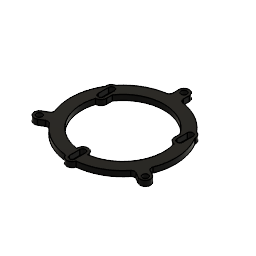
Mirror Mount Part 1 v1 (Autodesk Fusion 360 design; units mm, degrees)
Autodesk Fusion 360 part; units mm, degrees
note: some values were not read from the file. Set by a fixed rule: which sketch regions a step uses.
sketch "Sketch1" plane through (0, 0, 0) normal (0, 1, 0) x (1, 0, 0)
  circle A0 centre (0, 0) radius 26
  line L0 (0, 0) -> (22.5167, 13)
  line L1 (0, 0) -> (26, 0) construction
  line L2 (0, 0) -> (-22.5167, 13)
  line L3 (0, 0) -> (26, 0) construction
  line L4 (0, 0) -> (0, -26)
  circle A1 centre (0, 0) radius 23.5
  circle A2 centre (0, 0) radius 28.5
  line L5 (-22.5167, 13) -> (-22.5167, 16)
  line L6 (-22.5167, 13) -> (-22.5167, 10)
  line L7 (-24.1667, 10) -> (-24.1667, 16)
  line L8 (-20.8667, 10) -> (-20.8667, 16)
  line L9 (0, -26) -> (0, -23)
  line L10 (0, -26) -> (0, -29)
  line L11 (0, -26) -> (0, -23)
  line L12 (0, -29) -> (-1.65, -29)
  line L13 (-1.65, -29) -> (-1.65, -23)
  line L14 (1.65, -23) -> (1.65, -29)
  line L15 (24.1667, 10) -> (24.1667, 16)
  line L16 (20.8667, 10) -> (20.8667, 16)
  arc A3 (-1.65, -29) -> (1.65, -29) centre (0, -29) ccw
  arc A4 (1.65, -23) -> (-1.65, -23) centre (0, -23) ccw
  arc A5 (20.8667, 10) -> (24.1667, 10) centre (22.5167, 10) ccw
  arc A6 (24.1667, 16) -> (20.8667, 16) centre (22.5167, 16) ccw
  arc A7 (-24.1667, 10) -> (-20.8667, 10) centre (-22.5167, 10) ccw
  arc A8 (-20.8667, 16) -> (-24.1667, 16) centre (-22.5167, 16) ccw
  line L17 (-25.6667, 10) -> (-25.6667, 16)
  arc A9 (-19.3667, 16) -> (-25.6667, 16) centre (-22.5167, 16) ccw
  line L18 (-19.3667, 10) -> (-19.3667, 16)
  arc A10 (-25.6667, 10) -> (-19.3667, 10) centre (-22.5167, 10) ccw
  line L19 (-3.15, -29) -> (-3.15, -23)
  arc A11 (3.15, -23) -> (-3.15, -23) centre (0, -23) ccw
  line L20 (3.15, -23) -> (3.15, -29)
  arc A12 (-3.15, -29) -> (3.15, -29) centre (0, -29) ccw
  line L21 (19.3667, 10) -> (19.3667, 16)
  arc A13 (25.6667, 16) -> (19.3667, 16) centre (22.5167, 16) ccw
  line L22 (25.6667, 10) -> (25.6667, 16)
  arc A14 (19.3667, 10) -> (25.6667, 10) centre (22.5167, 10) ccw
  dimension "d1" = 52
  dimension "d2" = 30
  dimension "d3" = 150
  dimension "d7" = 47
  dimension "d8" = 57
  dimension "d9" = 3
  dimension "d11" = 3.3
  dimension "d12" = 3
  dimension "d13" = 3
  dimension "d14" = 3.3
  dimension "d15" = 3.3
  dimension "d23" = 1.5
  dimension "d24" = 1.5
  dimension "d25" = 1.5
  constraint coincident A0.centre L0.start
  constraint horizontal L1
  constraint horizontal L3
  constraint coincident A0 L4.end
  constraint perpendicular L1 L4
  constraint concentric A0 A1
  constraint concentric A0 A2
  constraint vertical L5
  constraint vertical L6
  constraint coincident L6.end A7.centre
  constraint vertical L8
  constraint coincident L4 L9.end
  constraint parallel L9 L10
  constraint parallel L4 L11
  constraint coincident L9.end L11.end
  constraint coincident L10.end L12.start
  constraint perpendicular L10 L12
  constraint tangent L13 A4
  constraint tangent L14 A3
  constraint parallel L13 L14
  constraint symmetric L4 A5 A7
  constraint symmetric L4 L7.start L15.start
  constraint symmetric L4 L7.end L15.end
  constraint symmetric L4 L8.start L16.start
  constraint symmetric L4 L8.end L16.end
  measures "d1" diameter of A0
  measures "d2" angle of L0 L1
  measures "d3" angle of L2 L3
  measures "d7" diameter of A1
  measures "d8" diameter of A2
  measures "d9" distance of L2.end L5.end
  measures "d11" diameter of A7
  measures "d12" distance of L4.end L10.end
  measures "d13" distance of L4.end L9.end
  measures "d14" diameter of A4
  measures "d15" diameter of A3
extrude "Extrude2" add sketch "Sketch1" along normal blind 3 contours A0 A1 L20 A14 | A0 A2 L20 L22 A14 | A0 A1 A5 A14 | A0 A2 L15 A5 L22 A14 | A0 A2 L14 L20 | A0 A1 L14 L20 | L0 A1 L16 A5 L21 A14 | L4 A1 L14 A4 A11 L20 | A2 L13 L14 A3 L19 L20 A12 | A2 L15 A6 A13 L22 | A0 L0 A1 L16 L21 A13 | A0 A2 L16 A6 A13 | L0 A1 L16 | L0 A1 L21 | A0 A2 L13 L19 | A0 A1 L13 L19 | L4 A1 L13 A4 L19 A11 | A0 A1 A9 L18 L21 A13 | A0 A2 A9 A13 | A0 A2 L17 A10 L19 | A0 A1 A10 L19 | A0 L2 A1 L8 A9 L18 | A0 A2 L8 A8 A9 | L2 A1 L8 A7 L18 A10 | L2 A1 L18 | A2 L7 A8 L17 A9 | A0 A2 L7 A7 L17 A10 | A0 A1 A7 A10 | L2 A1 L8
sketch "Sketch2" plane through (0, 3, 0) normal (0, 1, 0) x (-1, 0, 0)
  arc A0 (-20.8667, -10) -> (-24.1667, -10) centre (-22.5167, -10) ccw
  line L0 (-20.8667, -10) -> (-20.8667, -16)
  arc A1 (-24.1667, -16) -> (-20.8667, -16) centre (-22.5167, -16) ccw
  line L1 (-24.1667, -16) -> (-24.1667, -10)
  arc A2 (24.1667, -10) -> (20.8667, -10) centre (22.5167, -10) ccw
  line L2 (24.1667, -10) -> (24.1667, -16)
  arc A3 (20.8667, -16) -> (24.1667, -16) centre (22.5167, -16) ccw
  line L3 (20.8667, -16) -> (20.8667, -10)
  arc A4 (1.65, 29) -> (-1.65, 29) centre (0, 29) ccw
  line L4 (1.65, 29) -> (1.65, 23)
  arc A5 (-1.65, 23) -> (1.65, 23) centre (0, 23) ccw
  line L5 (-1.65, 23) -> (-1.65, 29)
  arc A6 (-19.3667, -13.311) -> (19.3667, -13.311) centre (0, 0) ccw
  line L6 (-19.3667, -13.311) -> (-19.3667, -10)
  arc A7 (-19.3667, -10) -> (-22.4794, -6.8502) centre (-22.5167, -10) ccw
  arc A8 (-3.15, 23.2879) -> (-22.4794, -6.8502) centre (0, 0) ccw
  line L7 (-3.15, 23.2879) -> (-3.15, 23)
  arc A9 (-3.15, 23) -> (3.15, 23) centre (0, 23) ccw
  line L8 (3.15, 23) -> (3.15, 23.2879)
  arc A10 (22.4794, -6.8502) -> (3.15, 23.2879) centre (0, 0) ccw
  arc A11 (22.4794, -6.8502) -> (19.3667, -10) centre (22.5167, -10) ccw
  line L9 (19.3667, -10) -> (19.3667, -13.311)
  arc A12 (3.15, 29) -> (-3.15, 29) centre (0, 29) ccw
  line L10 (-3.15, 29) -> (-3.15, 28.3254)
  arc A13 (-3.15, 28.3254) -> (-25.6667, -12.3884) centre (0, 0) ccw
  line L11 (-25.6667, -12.3884) -> (-25.6667, -16)
  arc A14 (-25.6667, -16) -> (-21.3196, -18.9137) centre (-22.5167, -16) ccw
  arc A15 (-21.3196, -18.9137) -> (21.3196, -18.9137) centre (0, 0) ccw
  arc A16 (21.3196, -18.9137) -> (25.6667, -16) centre (22.5167, -16) ccw
  line L12 (25.6667, -16) -> (25.6667, -12.3884)
  arc A17 (25.6667, -12.3884) -> (3.15, 28.3254) centre (0, 0) ccw
  line L13 (3.15, 28.3254) -> (3.15, 29)
  circle A18 centre (0, 0) radius 23.75
  circle A19 centre (0, 0) radius 30
  circle A20 centre (0, 0) radius 25 construction
  circle A21 centre (0, 0) radius 27.5 construction
  line L14 (0, 0) -> (0, -35)
  line L15 (0, 0) -> (-30.3109, 17.5)
  line L16 (0, 0) -> (35, 0) construction
  line L17 (0, 0) -> (30.3109, 17.5)
  line L18 (0, 0) -> (35, 0) construction
  circle A22 centre (30.3109, 17.5) radius 1.65
  circle A23 centre (-30.3109, 17.5) radius 1.65
  circle A24 centre (0, -35) radius 1.65
  circle A25 centre (0, -35) radius 3
  circle A26 centre (30.3109, 17.5) radius 3
  circle A27 centre (-30.3109, 17.5) radius 3
  line L19 (-30.3109, 17.5) -> (-31.8109, 14.9019)
  line L20 (-31.8109, 14.9019) -> (-27.3505, 12.3267)
  line L21 (-30.3109, 17.5) -> (-28.8109, 20.0981)
  line L22 (-28.8109, 20.0981) -> (-24.3505, 17.5229)
  line L23 (31.8109, 14.9019) -> (27.3505, 12.3267)
  line L24 (28.8109, 20.0981) -> (24.3505, 17.5229)
  line L25 (3, -35) -> (3, -29.8496)
  line L26 (0, -35) -> (3, -35)
  line L27 (0, -35) -> (-3, -35)
  line L28 (-3, -35) -> (-3, -29.8496)
  dimension "d28" = 47.5
  dimension "d29" = 60
  dimension "d32" = 50
  dimension "d33" = 55
  dimension "d39" = 35
  dimension "d40" = 150
  dimension "d41" = 35
  dimension "d42" = 35
  dimension "d43" = 30
  dimension "d44" = 3.3
  dimension "d45" = 3.3
  dimension "d46" = 3.3
  dimension "d47" = 6
  dimension "d48" = 6
  dimension "d49" = 6
  constraint coincident A6.centre A8.centre
  constraint concentric A19 A20
  constraint concentric A20 A21
  constraint vertical L14
  constraint horizontal L16
  constraint horizontal L18
  constraint coincident L17.end A22.centre
  constraint coincident L15.end A23.centre
  constraint coincident L14.end A24.centre
  constraint concentric A24 A25
  constraint concentric A22 A26
  constraint concentric A23 A27
  constraint coincident A27 L19.end
  constraint perpendicular L15 L19
  constraint coincident A19 L20.end
  constraint tangent A27 L20
  constraint coincident A27 L21.end
  constraint perpendicular L15 L21
  constraint coincident A19 L22.end
  constraint tangent A27 L22
  constraint coincident A26 L23.start
  constraint coincident A19 L23.end
  constraint tangent A26 L23
  constraint coincident A26 L24.start
  constraint coincident A19 L24.end
  constraint tangent A26 L24
  constraint parallel L23 L24
  constraint coincident A25 L25.start
  constraint coincident A19 L25.end
  constraint vertical L25
  constraint coincident A25 L27.end
  constraint parallel L26 L27
  constraint coincident A19 L28.end
  constraint perpendicular L27 L28
  measures "d28" diameter of A18
  measures "d29" diameter of A19
  measures "d32" diameter of A20
  measures "d33" diameter of A21
  measures "d39" distance of A6.centre L14.end
  measures "d40" angle of L15 L16
  measures "d41" distance of A6.centre L15.end
  measures "d42" distance of A6.centre L17.end
  measures "d43" angle of L17 L18
  measures "d44" diameter of A22
  measures "d45" diameter of A23
  measures "d46" diameter of A24
  measures "d47" diameter of A25
  measures "d48" diameter of A26
  measures "d49" diameter of A27
extrude "Extrude3" add sketch "Sketch2" against normal blind 3 contours A12 L10 A13 A19 L15 | A13 L11 A19 L15 | A14 A15 A19 L14 | A15 A16 A19 L14 | A19 L15 A27 L22 | A19 L15 A27 L20 | A19 L14 A25 L28 | A19 L14 A25 L25 | L15 A23 A27 L19 | L15 A23 A27 L21 | L14 A24 A25 L26 | L14 A24 A25 L27 | L12 A17 A19 L17 | A12 A17 L13 A19 L17 | A23 A27 L19 L21 | A24 A25 L26 L27 | A19 L17 A26 L23 | A19 L17 A26 L24 | A26
fillet "Fillet1" radius 2 6 edges at (-24.3505, 1.5, 17.5229) (-27.3505, 1.5, 12.3267) (-3, 1.5, -29.8496) (3, 1.5, -29.8496) (27.3505, 1.5, 12.3267) (24.3505, 1.5, 17.5229)
equation "d1 = ( 26 * 2 ) * 1 mm"
equation "d8 = 52 mm + 5 mm"
